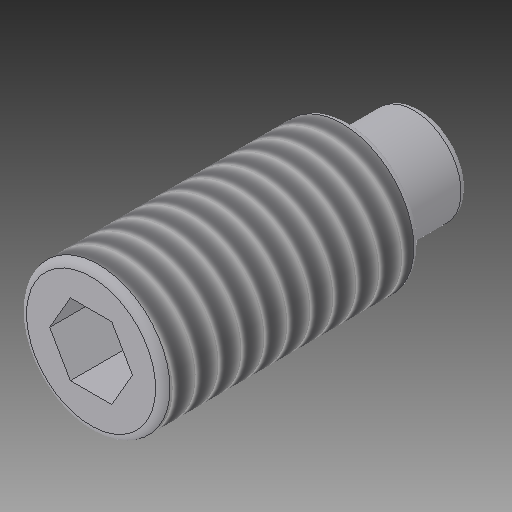
# Autodesk Inventor part: M5 pour ressort
Saved by Autodesk Inventor 2017 (Build 210142000, 142)
## iProperties
Company: FABLAB Frenchmakers
Part Number: M5 pour ressort
Material: ----------
Document SubType Name: Modeling
Designer: FABLAB Frenchmakers
Density: 7.86 g/cm^3
Appearance: Métal - Acier
Mass: 1.44639 g
Surface Area: 2.23644 cm^2
Volume: 0.184019 cm^3
Project: 1420 Vauban 3D XL
Catalog Web Link: http://frenchmakers.com/
Stock Number: 1420-05-21
Autodesk Inventor part; units mm, degrees
ref_plane "YZ Plane" through (0, 0, 0) normal (1, 0, 0) x (0, 1, 0)
ref_plane "XZ Plane" through (0, 0, 0) normal (0, 1, 0) x (-1, 0, 0)
ref_plane "XY Plane" through (0, 0, 0) normal (0, 0, 1) x (1, 0, 0)
sketch "Esquisse1" plane through (0, 0, 0) normal (0, 0, 1) x (1, 0, 0)
  circle A0 centre (0, 0) radius 2.5
  dimension "d0" = 5
  constraints: 1 centre point, 1 coincident
  measures "d0" diameter of A0
extrude "Extrusion1" add sketch "Esquisse1" along normal blind 9
sketch "Esquisse2" plane through (0, 0, 0) normal (0, 0, -1) x (-1, 0, 0)
  circle A0 centre (0, 0) radius 2.5 projected
  circle A1 centre (0, 0) radius 1.65
  dimension "d3" = 3.3
  constraints: 1 centre point, 1 coincident
  measures "d3" diameter of A1
extrude "Extrusion2" add sketch "Esquisse2" along normal blind 2.5 contours A1
thread "Filetage1" size "M5x0.8" class "6g" standard "ANSI Metric M Profile" full length
sketch "Esquisse3" plane through (0, 0, 9) normal (0, 0, 1) x (1, 0, 0)
  line L0 (0.7217, 1.25) -> (1.4434, 0)
  line L1 (1.4434, 0) -> (0.7217, -1.25)
  line L2 (0.7217, -1.25) -> (-0.7217, -1.25)
  line L3 (-0.7217, -1.25) -> (-1.4434, 0)
  line L4 (-1.4434, 0) -> (-0.7217, 1.25)
  line L5 (-0.7217, 1.25) -> (0.7217, 1.25)
  point P0 (0, 0)
  point P1 (0, 0)
  dimension "d8" = 2.5
  constraints: 12 end point, 1 coincident, 1 horizontal, 13 other
  measures "d8" distance between parallel lines of L2 L5
extrude "Extrusion3" cut sketch "Esquisse3" against normal blind 2.5
fillet "Congé1" radius 0.25 3 edges at (-2.5, 0, 9) (-2.5, 0, 0) (1.65, 0, -2.5)
